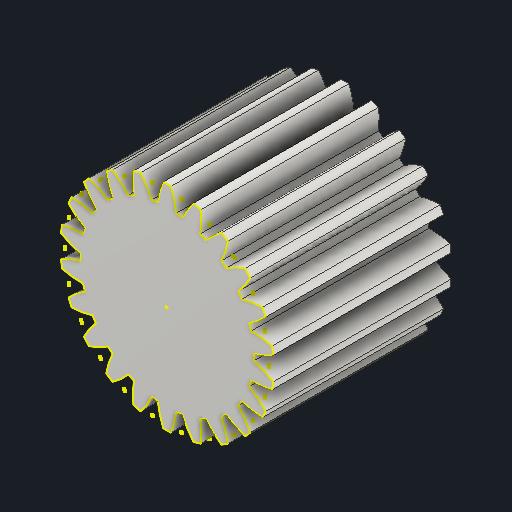
# Autodesk Inventor part: Цилиндрическое зубчатое зацепление2
Saved by Autodesk Inventor 2025 (Build 290162000, 162)
## iProperties
Created: 2025-01-03
Part Number: Цилиндрическое зубчатое зацепление2
Material: Steel
Document SubType Name: Modeling
Designer: GameHD
Categories: <?xml version="1.0" encoding="UTF-16"?> <MemberInstance><Categories><FamilyTemplate><FamilyTemplateParameter ValueType="xs:double" Id="1" ObjectReferenceKey="da_z" ObjectType="kUserParameterObject"/><FamilyTemplateParameter ValueType="xs:double" Id="2" ObjectReferenceKey="da_b" ObjectType="kUserParameterObject"/><FamilyTemplateParameter ValueType="xs:double" Id="3" ObjectReferenceKey="da_beta" ObjectType="kUserParameterObject"/><FamilyTemplateParameter ValueType="xs:double" Id="4" ObjectReferenceKey="da_da" ObjectType="kUserParameterObject"/><FamilyTemplateParameter ValueType="xs:double" Id="5" ObjectReferenceKey="da_aw" ObjectType="kUserParameterObject"/><FamilyTemplateParameter ValueType="xs:string" Id="6" ObjectReferenceKey="EAIAABAAAAC/AAAAAAAAAIAAAAAAAAAA" ObjectType="83910656" SubObjectId="SurfaceGeometry"/></FamilyTemplate><ParamToTemplateMap><ParamToTemplate CategoryParameter="//CategoryParameter[@InternalName='046C89C9-8512-4d59-83FE-43B91F4F132A']" TemplateParameter="1"/><ParamToTemplate CategoryParameter="//CategoryParameter[@InternalName='2552DF32-E462-4b46-AEBF-C6C7768E72AC']" TemplateParameter="2"/><ParamToTemplate CategoryParameter="//CategoryParameter[@InternalName='C9EE641D-15FC-4fae-A226-E94C4372FDD7']" TemplateParameter="3"/><ParamToTemplate><ParamToTemplate CategoryParameter="//CategoryParameter[@InternalName='00B6519A-459B-49c7-AD84-2E56D39A5744']" ConstantValue="0.000000"/></ParamToTemplate><ParamToTemplate><ParamToTemplate CategoryParameter="//CategoryParameter[@InternalName='04B31F0E-C7A6-4894-AA32-9629BEFACF47']" ConstantValue="1.000000"/></ParamToTemplate><ParamToTemplate><ParamToTemplate CategoryParameter="//CategoryParameter[@InternalName='43CBEC2E-7847-49e7-A936-2F7889FCB2D9']" ConstantValue="0.250000"/></ParamToTemplate><ParamToTemplate><ParamToTemplate CategoryParameter="//CategoryParameter[@InternalName='B1EFC894-105D-4ebd-86BF-FA20ED196853']" ConstantValue="0.350000"/></ParamToTemplate><ParamToTemplate><ParamToTemplate CategoryParameter="//CategoryParameter[@InternalName='51175063-3D10-4879-93E8-6246FE8B403D']" ConstantValue="2061532430.657340"/></ParamToTemplate><ParamToTemplate><ParamToTemplate CategoryParameter="//CategoryParameter[@InternalName='A3A52E27-4454-46a9-B0BD-C932399B70AF']" ConstantValue="0.300000"/></ParamToTemplate><ParamToTemplate><ParamToTemplate CategoryParameter="//CategoryParameter[@InternalName='91B76062-C214-41d9-B1B9-14D2AB99603D']" ConstantValue="0.127000"/></ParamToTemplate><ParamToTemplate><ParamToTemplate CategoryParameter="//CategoryParameter[@InternalName='374E806E-8B8A-4dda-A9AA-1039D6500AD2']" ConstantValue="7.874016"/></ParamToTemplate><ParamToTemplate><ParamToTemplate CategoryParameter="//CategoryParameter[@InternalName='2D373A89-B862-43d6-8D0B-0CBF12AB9F6C']" ConstantValue="0.349066"/></ParamToTemplate><ParamToTemplate CategoryParameter="//CategoryParameter[@InternalName='37777632-D6A2-4fac-9D53-DB8ACD95C989']" TemplateParameter="4"/><ParamToTemplate CategoryParameter="//CategoryParameter[@InternalName='FD1017F1-B727-4f7e-9707-0F86F1FF9423']" TemplateParameter="5"/><ParamToTemplate><ParamToTemplate CategoryParameter="//CategoryParameter[@InternalName='9E1B4470-B2D3-4ff1-B813-535BB4CDF51A']" ConstantValue="3523220.976809"/></ParamToTemplate><ParamToTemplate><ParamToTemplate CategoryParameter="//CategoryParameter[@InternalName='F8452263-BFF6-458c-9FB1-07C4B99E95CD']" ConstantValue="11397033.805607"/></ParamToTemplate><ParamToTemplate><ParamToTemplate CategoryParameter="//CategoryParameter[@InternalName='3E3BB259-FD49-497f-8171-6EBC954A3479']" ConstantValue="2.000000"/></ParamToTemplate><ParamToTemplate CategoryParameter="//CategoryParameter[@InternalName='27C3BAF2-7550-4e4b-AE2C-0DB134B7D9B7']" TemplateParameter="6"/></ParamToTemplateMap><Category DisplayName="Gear" InternalName="DC85795E-93AB-48d5-8EEE-5A27447B64BD" Mnemonic="Gear"><CategoryParameter DisplayName="z" InternalName="046C89C9-8512-4d59-83FE-43B91F4F132A" Mnemonic="z"/><CategoryParameter DisplayName="b" InternalName="2552DF32-E462-4b46-AEBF-C6C7768E72AC" Mnemonic="b"/><CategoryParameter DisplayName="||b|" InternalName="C9EE641D-15FC-4fae-A226-E94C4372FDD7" Mnemonic="beta"/><CategoryParameter DisplayName="x" InternalName="00B6519A-459B-49c7-AD84-2E56D39A5744" Mnemonic="x"/><CategoryParameter DisplayName="a*" InternalName="04B31F0E-C7A6-4894-AA32-9629BEFACF47" Mnemonic="a"/><CategoryParameter DisplayName="c*" InternalName="43CBEC2E-7847-49e7-A936-2F7889FCB2D9" Mnemonic="c"/><CategoryParameter DisplayName="r|.f|*" InternalName="B1EFC894-105D-4ebd-86BF-FA20ED196853" Mnemonic="rf"/><CategoryParameter DisplayName="E" InternalName="51175063-3D10-4879-93E8-6246FE8B403D" Mnemonic="E"/><CategoryParameter DisplayName="||m|" InternalName="A3A52E27-4454-46a9-B0BD-C932399B70AF" Mnemonic="mi"/><Category DisplayName="SpurGear" InternalName="26C5A22E-A91E-4dfd-A3B3-23CCAFAE1764" Mnemonic="SpurGear"><CategoryParameter DisplayName="m" InternalName="91B76062-C214-41d9-B1B9-14D2AB99603D" Mnemonic="m"/><CategoryParameter DisplayName="P" InternalName="374E806E-8B8A-4dda-A9AA-1039D6500AD2" Mnemonic="PP"/><CategoryParameter DisplayName="||a|" InternalName="2D373A89-B862-43d6-8D0B-0CBF12AB9F6C" Mnemonic="alpha"/><CategoryParameter DisplayName="d|.a|" InternalName="37777632-D6A2-4fac-9D53-DB8ACD95C989" Mnemonic="da"/><CategoryParameter DisplayName="a|.w|" InternalName="FD1017F1-B727-4f7e-9707-0F86F1FF9423" Mnemonic="aw"/><CategoryParameter DisplayName="||s||.Flim|" InternalName="9E1B4470-B2D3-4ff1-B813-535BB4CDF51A" Mnemonic="sFlim"/><CategoryParameter DisplayName="||s||.Hlim|" InternalName="F8452263-BFF6-458c-9FB1-07C4B99E95CD" Mnemonic="sHlim"/><CategoryParameter DisplayName="тип" InternalName="3E3BB259-FD49-497f-8171-6EBC954A3479" Mnemonic="type"/><CategoryParameter DisplayName="PitchDiameter" InternalName="27C3BAF2-7550-4e4b-AE2C-0DB134B7D9B7" Mnemonic="IDS_PITCHDIAM"/></Category></Category></Categories></MemberInstance>
Density: 1 g/cm^3
Appearance: Steel
CustomPartVersion: 1
Author: GameHD
Autodesk Inventor part; units mm, degrees
sketch "Sketch1" plane through (0, 0, 0) normal (0, 0, 1) x (1, 0, 0)
  circle A0 centre (0, 0) radius 15.24
  dimension "d0" = 30.48
  constraints: 1 centre point
  measures "d0" diameter of A0
extrude "Extrusion1" add sketch "Sketch1" along normal blind 25.4
sketch "Sketch2" plane through (0, 0, 0) normal (0, 0, -1) x (-1, 0, 0)
  circle A0 centre (0, 0) radius 15.24 projected
  circle A1 centre (0, 0) radius 13.97
  dimension "d3" = 27.94
  constraints: 1 centre point, 1 coincident
  measures "d3" diameter of A1
surface extrude "Средний диаметр" sketch "Sketch2" against normal through all shown no curves A1
ref_plane "Work Plane1" through (0, 0, 0) normal (1, 0, 0) x (0, 1, 0)
ref_plane "Work Plane2" through (0, 0, 0) normal (0.9898214, 0.1423148, 0) x (0, 0, 1)
ref_plane "Work Plane3" through (0, 0, 12.7) normal (0, 0, -1) x (-1, 0, 0)
spur gear teeth "Цилиндрическое зубчатое зацепление" teeth 22 pitch diameter 27.94 tip diameter 30.48 root diameter 24.765 face width 25.4 start plane through (0, 0, 0) normal (0, 0, -1) x (-1, 0, 0)
sketch "Эскиз3" plane through (0, 0, 25.4) normal (0, 0, 1) x (1, 0, 0)
  arc A0 (-4.8128, 14.4601) -> (-4.7386, 11.4399) centre (6.161, 13.2187) ccw projected
  arc A1 (-4.7386, 11.4399) -> (-5.5426, 11.0727) centre (0, 0) ccw projected
  arc A2 (-5.5426, 11.0727) -> (-7.7765, 13.1066) centre (-14.0246, 4.0003) ccw projected
  arc A3 (-7.7765, 13.1066) -> (-8.6917, 12.5185) centre (0, 0) ccw projected
  arc A4 (-8.6917, 12.5185) -> (-7.7696, 9.6415) centre (2.1873, 14.419) ccw projected
  arc A5 (-7.7696, 9.6415) -> (-8.4377, 9.0627) centre (0, 0) ccw projected
  arc A6 (-8.4377, 9.0627) -> (-11.1541, 10.3848) centre (-14.5836, -0.1129) ccw projected
  arc A7 (-11.1541, 10.3848) -> (-11.8665, 9.5626) centre (0, 0) ccw projected
  arc A8 (-11.8665, 9.5626) -> (-10.1712, 7.062) centre (-1.9637, 14.4512) ccw projected
  arc A9 (-10.1712, 7.062) -> (-10.6491, 6.3184) centre (0, 0) ccw projected
  arc A10 (-10.6491, 6.3184) -> (-13.628, 6.8217) centre (-13.961, -4.217) ccw projected
  arc A11 (-13.628, 6.8217) -> (-14.0799, 5.8321) centre (0, 0) ccw projected
  arc A12 (-14.0799, 5.8321) -> (-11.7488, 3.9104) centre (-5.9555, 13.3126) ccw projected
  arc A13 (-11.7488, 3.9104) -> (-11.9979, 3.0623) centre (0, 0) ccw projected
  arc A14 (-11.9979, 3.0623) -> (-14.9979, 2.7059) centre (-12.2074, -7.9795) ccw projected
  arc A15 (-14.9979, 2.7059) -> (-15.1527, 1.6291) centre (0, 0) ccw projected
  arc A16 (-15.1527, 1.6291) -> (-12.3746, 0.442) centre (-9.4648, 11.0955) ccw projected
  arc A17 (-12.3746, 0.442) -> (-12.3746, -0.442) centre (0, 0) ccw projected
  arc A18 (-12.3746, -0.442) -> (-15.1527, -1.6291) centre (-9.4648, -11.0955) ccw projected
  arc A19 (-15.1527, -1.6291) -> (-14.9979, -2.7059) centre (0, 0) ccw projected
  arc A20 (-14.9979, -2.7059) -> (-11.9979, -3.0623) centre (-12.2074, 7.9795) ccw projected
  arc A21 (-11.9979, -3.0623) -> (-11.7488, -3.9104) centre (0, 0) ccw projected
  arc A22 (-11.7488, -3.9104) -> (-14.0799, -5.8321) centre (-5.9555, -13.3126) ccw projected
  arc A23 (-14.0799, -5.8321) -> (-13.628, -6.8217) centre (0, 0) ccw projected
  arc A24 (-13.628, -6.8217) -> (-10.6491, -6.3184) centre (-13.961, 4.217) ccw projected
  arc A25 (-10.6491, -6.3184) -> (-10.1712, -7.062) centre (0, 0) ccw projected
  arc A26 (-10.1712, -7.062) -> (-11.8665, -9.5626) centre (-1.9637, -14.4512) ccw projected
  arc A27 (-11.8665, -9.5626) -> (-11.1541, -10.3848) centre (0, 0) ccw projected
  arc A28 (-11.1541, -10.3848) -> (-8.4377, -9.0627) centre (-14.5836, 0.1129) ccw projected
  arc A29 (-8.4377, -9.0627) -> (-7.7696, -9.6415) centre (0, 0) ccw projected
  arc A30 (-7.7696, -9.6415) -> (-8.6917, -12.5185) centre (2.1873, -14.419) ccw projected
  arc A31 (-8.6917, -12.5185) -> (-7.7765, -13.1066) centre (0, 0) ccw projected
  arc A32 (-7.7765, -13.1066) -> (-5.5426, -11.0727) centre (-14.0246, -4.0003) ccw projected
  arc A33 (-5.5426, -11.0727) -> (-4.7386, -11.4399) centre (0, 0) ccw projected
  arc A34 (-4.7386, -11.4399) -> (-4.8128, -14.4601) centre (6.161, -13.2187) ccw projected
  arc A35 (-4.8128, -14.4601) -> (-3.769, -14.7666) centre (0, 0) ccw projected
  arc A36 (-3.769, -14.7666) -> (-2.1986, -12.1858) centre (-12.3295, -7.7894) ccw projected
  arc A37 (-2.1986, -12.1858) -> (-1.3236, -12.3116) centre (0, 0) ccw projected
  arc A38 (-1.3236, -12.3116) -> (-0.544, -15.2303) centre (9.6356, -10.9475) ccw projected
  arc A39 (-0.544, -15.2303) -> (0.544, -15.2303) centre (0, 0) ccw projected
  arc A40 (0.544, -15.2303) -> (1.3236, -12.3116) centre (-9.6356, -10.9475) ccw projected
  arc A41 (1.3236, -12.3116) -> (2.1986, -12.1858) centre (0, 0) ccw projected
  arc A42 (2.1986, -12.1858) -> (3.769, -14.7666) centre (12.3295, -7.7894) ccw projected
  arc A43 (3.769, -14.7666) -> (4.8128, -14.4601) centre (0, 0) ccw projected
  arc A44 (4.8128, -14.4601) -> (4.7386, -11.4399) centre (-6.161, -13.2187) ccw projected
  arc A45 (4.7386, -11.4399) -> (5.5426, -11.0727) centre (0, 0) ccw projected
  arc A46 (5.5426, -11.0727) -> (7.7765, -13.1066) centre (14.0246, -4.0003) ccw projected
  arc A47 (7.7765, -13.1066) -> (8.6917, -12.5185) centre (0, 0) ccw projected
  arc A48 (8.6917, -12.5185) -> (7.7696, -9.6415) centre (-2.1873, -14.419) ccw projected
  arc A49 (7.7696, -9.6415) -> (8.4377, -9.0627) centre (0, 0) ccw projected
  arc A50 (8.4377, -9.0627) -> (11.1541, -10.3848) centre (14.5836, 0.1129) ccw projected
  arc A51 (11.1541, -10.3848) -> (11.8665, -9.5626) centre (0, 0) ccw projected
  arc A52 (11.8665, -9.5626) -> (10.1712, -7.062) centre (1.9637, -14.4512) ccw projected
  arc A53 (10.1712, -7.062) -> (10.6491, -6.3184) centre (0, 0) ccw projected
  arc A54 (10.6491, -6.3184) -> (13.628, -6.8217) centre (13.961, 4.217) ccw projected
  arc A55 (13.628, -6.8217) -> (14.0799, -5.8321) centre (0, 0) ccw projected
  arc A56 (14.0799, -5.8321) -> (11.7488, -3.9104) centre (5.9555, -13.3126) ccw projected
  arc A57 (11.7488, -3.9104) -> (11.9979, -3.0623) centre (0, 0) ccw projected
  arc A58 (11.9979, -3.0623) -> (14.9979, -2.7059) centre (12.2074, 7.9795) ccw projected
  arc A59 (14.9979, -2.7059) -> (15.1527, -1.6291) centre (0, 0) ccw projected
  arc A60 (15.1527, -1.6291) -> (12.3746, -0.442) centre (9.4648, -11.0955) ccw projected
  arc A61 (12.3746, -0.442) -> (12.3746, 0.442) centre (0, 0) ccw projected
  arc A62 (12.3746, 0.442) -> (15.1527, 1.6291) centre (9.4648, 11.0955) ccw projected
  arc A63 (15.1527, 1.6291) -> (14.9979, 2.7059) centre (0, 0) ccw projected
  arc A64 (14.9979, 2.7059) -> (11.9979, 3.0623) centre (12.2074, -7.9795) ccw projected
  arc A65 (11.9979, 3.0623) -> (11.7488, 3.9104) centre (0, 0) ccw projected
  arc A66 (11.7488, 3.9104) -> (14.0799, 5.8321) centre (5.9555, 13.3126) ccw projected
  arc A67 (14.0799, 5.8321) -> (13.628, 6.8217) centre (0, 0) ccw projected
  arc A68 (13.628, 6.8217) -> (10.6491, 6.3184) centre (13.961, -4.217) ccw projected
  arc A69 (10.6491, 6.3184) -> (10.1712, 7.062) centre (0, 0) ccw projected
  arc A70 (10.1712, 7.062) -> (11.8665, 9.5626) centre (1.9637, 14.4512) ccw projected
  arc A71 (11.8665, 9.5626) -> (11.1541, 10.3848) centre (0, 0) ccw projected
  arc A72 (11.1541, 10.3848) -> (8.4377, 9.0627) centre (14.5836, -0.1129) ccw projected
  arc A73 (8.4377, 9.0627) -> (7.7696, 9.6415) centre (0, 0) ccw projected
  arc A74 (7.7696, 9.6415) -> (8.6917, 12.5185) centre (-2.1873, 14.419) ccw projected
  arc A75 (8.6917, 12.5185) -> (7.7765, 13.1066) centre (0, 0) ccw projected
  arc A76 (7.7765, 13.1066) -> (5.5426, 11.0727) centre (14.0246, 4.0003) ccw projected
  arc A77 (5.5426, 11.0727) -> (4.7386, 11.4399) centre (0, 0) ccw projected
  arc A78 (4.7386, 11.4399) -> (4.8128, 14.4601) centre (-6.161, 13.2187) ccw projected
  arc A79 (4.8128, 14.4601) -> (3.769, 14.7666) centre (0, 0) ccw projected
  arc A80 (3.769, 14.7666) -> (2.1986, 12.1858) centre (12.3295, 7.7894) ccw projected
  arc A81 (2.1986, 12.1858) -> (1.3236, 12.3116) centre (0, 0) ccw projected
  arc A82 (1.3236, 12.3116) -> (0.544, 15.2303) centre (-9.6356, 10.9475) ccw projected
  arc A83 (0.544, 15.2303) -> (-0.544, 15.2303) centre (0, 0) ccw projected
  arc A84 (-0.544, 15.2303) -> (-1.3236, 12.3116) centre (9.6356, 10.9475) ccw projected
  arc A85 (-1.3236, 12.3116) -> (-2.1986, 12.1858) centre (0, 0) ccw projected
  arc A86 (-2.1986, 12.1858) -> (-3.769, 14.7666) centre (-12.3295, 7.7894) ccw projected
  arc A87 (-3.769, 14.7666) -> (-4.8128, 14.4601) centre (0, 0) ccw projected
equation "\"d0\" = da_da"
equation "\"d1\" = da_b"
equation "\"d3\" = da_d"
equation "\"d15\" = da_aw"
equation "\"d19\" = da_aw"
equation "\"da_da\" = 30.48"
equation "\"da_b\" = 25.4"
equation "\"da_d\" = 27.94"
equation "\"da_aw\" = 34.29"
body "Solid1"
body "Srf1"
